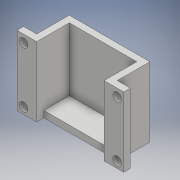
# Autodesk Inventor part: AprieteEthernet
Saved by Autodesk Inventor 2017 (Build 210142000, 142)
## iProperties
Created: 2021-08-13
Part Number: AprieteEthernet
Material: Generic
Document SubType Name: Modeling
Designer: USUARIO
Density: 1 g/cm^3
Appearance: Default
Author: USUARIO
Autodesk Inventor part; units mm, degrees
ref_plane "YZ Plane" through (0, 0, 0) normal (1, 0, 0) x (0, 1, 0)
ref_plane "XZ Plane" through (0, 0, 0) normal (0, 1, 0) x (-1, 0, 0)
ref_plane "XY Plane" through (0, 0, 0) normal (0, 0, 1) x (1, 0, 0)
sketch "Sketch1" plane through (0, 0, 0) normal (0, 1, 0) x (-1, 0, 0)
  line L0 (0, 0) -> (31, 0)
  line L1 (31, 0) -> (31, -32)
  line L2 (31, -32) -> (0, -32)
  line L3 (0, -32) -> (0, 0)
  dimension "d0" = 31
  dimension "d1" = 32
  constraints: 8 end point, 2 parallel, 1 horizontal, 1 perpendicular
  measures "d0" distance of L1.end L2.end
  measures "d1" distance of L0.end L1.end
extrude "Extrusion1" add sketch "Sketch1" along normal blind 3
sketch "Sketch2" plane through (-31, 0, -32) normal (-1, 0, 0) x (0, 0, 1)
  line L0 (32, 3) -> (0, 3)
  line L1 (0, 3) -> (0, -15)
  line L2 (0, -15) -> (32, -15)
  line L3 (32, -15) -> (32, 3)
  point P0 (32, 0)
  dimension "d4" = 32
  dimension "d5" = 18
  constraints: 8 end point, 2 parallel, 1 horizontal, 1 perpendicular
  measures "d4" distance of L2.end L1.end
  measures "d5" distance of L1.end L0.end
extrude "Extrusion2" add sketch "Sketch2" along normal blind 3
sketch "Sketch3" plane through (0, 0, 0) normal (1, 0, 0) x (0, 0, -1)
  line L0 (0, 3) -> (32, 3)
  line L1 (32, 3) -> (32, -15)
  line L2 (32, -15) -> (0, -15)
  line L3 (0, -15) -> (0, 3)
  point P0 (0, 0)
  dimension "d8" = 32
  dimension "d9" = 18
  constraints: 8 end point, 2 parallel, 1 horizontal, 1 perpendicular
  measures "d8" distance of L1.end L2.end
  measures "d9" distance of L0.end L1.end
extrude "Extrusion3" add sketch "Sketch3" along normal blind 3
sketch "Sketch4" plane through (3, 0, 0) normal (1, 0, 0) x (0, 0, -1)
  line L0 (0, 3) -> (0, -15) projected
  line L1 (0, -15) -> (32, -15)
  line L2 (32, -15) -> (32, -12)
  line L3 (32, -12) -> (0, -12)
  line L4 (0, -12) -> (0, -15)
  point P0 (0, 0)
  dimension "d12" = 32
  dimension "d13" = 3
  constraints: 8 end point, 2 parallel, 1 horizontal, 1 perpendicular
  measures "d12" distance of L3.end L2.end
  measures "d13" distance of L2.end L1.end
extrude "Extrusion4" add sketch "Sketch4" along normal blind 6
sketch "Sketch5" plane through (-34, 0, -32) normal (-1, 0, 0) x (0, 0, 1)
  line L0 (0, -15) -> (32, -15) projected
  line L1 (0, -15) -> (32, -15)
  line L2 (32, -15) -> (32, -12)
  line L3 (32, -12) -> (0, -12)
  line L4 (0, -12) -> (0, -15)
  point P0 (32, 0)
  dimension "d16" = 32
  dimension "d17" = 3
  constraints: 8 end point, 2 parallel, 1 horizontal, 1 perpendicular
  measures "d16" distance of L3.end L2.end
  measures "d17" distance of L2.end L1.end
extrude "Extrusion5" add sketch "Sketch5" along normal blind 6
sketch "Sketch6" plane through (-34, -12, 0) normal (0, 1, 0) x (1, 0, 0)
  circle A0 centre (40, 28.97) radius 2
  circle A1 centre (40, 3.5) radius 2
  circle A2 centre (-3, 28.97) radius 2
  circle A3 centre (-3, 3.5) radius 2
  line L0 (37, 0) -> (43, 0) projected
  line L1 (0, 0) -> (-6, 0) projected
  line L2 (43, 32) -> (43, 0) projected
  line L3 (-6, 0) -> (-6, 32) projected
  point P0 (34, 0)
  dimension "d20" = 4
  dimension "d21" = 4
  dimension "d22" = 4
  dimension "d23" = 4
  dimension "d24" = 25.47
  dimension "d25" = 25.47
  dimension "d26" = 3.5
  dimension "d27" = 3.5
  dimension "d28" = 3
  dimension "d29" = 3
  dimension "d30" = 3
  constraints: 4 centre point
  measures "d20" diameter of A0
  measures "d21" diameter of A1
  measures "d22" diameter of A2
  measures "d23" diameter of A3
  measures "d24" distance of A1.centre A0.centre
  measures "d25" distance of A3.centre A2.centre
  measures "d26" distance from line of L0 A1.centre
  measures "d27" distance from line of L1 A3.centre
  measures "d28" distance from line of A0.centre L2
  measures "d29" distance from line of A2.centre L3
  measures "d30" distance from line of A3.centre L3
extrude "Extrusion6" cut sketch "Sketch6" against normal blind 6
sketch "Sketch7" plane through (0, 0, 0) normal (0, -1, 0) x (1, 0, 0)
  line L0 (0, -32) -> (9, -32) projected
  line L1 (-31, -32) -> (-31, 0) projected
  line L2 (0, -32) -> (-31, -32)
  line L3 (-31, -32) -> (-31, -29)
  line L4 (-31, -29) -> (0, -29)
  line L5 (0, -29) -> (0, -32)
  point P0 (0, 0)
  dimension "d33" = 3
  constraints: 8 end point, 2 parallel, 1 horizontal, 1 perpendicular, 1 point on line
  measures "d33" distance of L2.end L3.end
extrude "Extrusion7" add sketch "Sketch7" along normal blind 11.7
body "Solid1"
